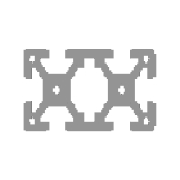
# Autodesk Inventor part: 615 mm
Saved by Autodesk Inventor 2016 (Build 200138000, 138)
## iProperties
IsCustomPart: 1
Created: 2023-12-03
Part Number: 615 mm
Material: Aluminum 6061
Description: ALU PROFILE 3060
Document SubType Name: Modeling
Standard: ALU PROFILE 3060
Designer: Riskinova Oktavia
Standard Revision: ALU PROFILE 3060
Manufacturer: ALU PROFILE 3060
Standards Organization: ALU PROFILE 3060
Language: en-US
Size Designation: (Unnamed 1)
Categories: <MemberInstance><Categories><Category DisplayName="Structural Shapes" InternalName="089c4875-fa83-4c05-b084-43b9cc11f5ed" Mnemonic="GRDR"><CategoryParameter DisplayName="Mass per Length Unit" InternalName="0bb95a10-148f-4027-a459-38d7b056702a" Mnemonic="shpmass"/><CategoryParameter DisplayName="Section Area" InternalName="1ff91680-64b0-4202-b9a3-7fd3f94bba3b" Mnemonic="secarea"/><CategoryParameter DisplayName="Radius of Gyration (x)" InternalName="25778675-03e9-40c1-b6a8-4a9ed693320d" Mnemonic="gyrradx"/><CategoryParameter DisplayName="Torsional Rigidity Modulus" InternalName="26c1ec35-5026-4c63-ad0a-751cf684a536" Mnemonic="torrigmod"/><CategoryParameter DisplayName="Distance of the Center of Gravity X-X" InternalName="26c9bdb8-9c79-4b4f-a92e-8e197583c9c4" Mnemonic="grcendistX"/><CategoryParameter DisplayName="Legacy Member ID" InternalName="340afe4f-75d7-48d3-ab7d-943f3c3da468" Mnemonic="LegacyMemberID"/><CategoryParameter DisplayName="Base Length" InternalName="42e34263-8f20-4d0e-ad48-bf1385b87c24" Mnemonic="shplen"/><CategoryParameter DisplayName="Moment of Inertia (y)" InternalName="4b9f58ea-bced-460e-81ea-3d29ca5a49e3" Mnemonic="inermomy"/><CategoryParameter DisplayName="Moment of Inertia (x)" InternalName="4cd780bc-73d7-43ac-917a-579e5cbd684d" Mnemonic="inermomx"/><CategoryParameter DisplayName="Custom Base Point" InternalName="4f1d1b73-316d-484b-a3df-9cbabb16eb77" Mnemonic="shpBasePoint"/><CategoryParameter DisplayName="Shape Height" InternalName="50274e7d-5ac0-4796-92cb-c59e54983c67" Mnemonic="shpheig"/><CategoryParameter DisplayName="Section Module (y)" InternalName="59eaa5e9-d227-48dc-b6c1-6920f96e0f95" Mnemonic="secmody"/><CategoryParameter DisplayName="Section Designation" InternalName="5a64d034-428d-49c8-ba32-7619764de20f" Mnemonic="shpdes"/><CategoryParameter DisplayName="Section Module (x)" InternalName="72cfad18-cf51-4ed4-aaa7-c6b224f8419f" Mnemonic="secmodx"/><CategoryParameter DisplayName="Torsional Section Modulus" InternalName="7c55a8dc-8844-49f9-a867-cc677b30ec9a" Mnemonic="torsecmod"/><CategoryParameter DisplayName="Shape Width" InternalName="7c717d54-a18f-4666-b4d4-573cce22c62c" Mnemonic="shpwdth"/><CategoryParameter DisplayName="Second Shape Thickness" InternalName="9251a8e1-85fd-4e47-af99-afdb762317d9" Mnemonic="shpthick2"/><CategoryParameter DisplayName="FG Authored" InternalName="9c666724-f362-4ea7-ac62-f6a007de5c69" Mnemonic="shpFGAuto"/><CategoryParameter DisplayName="Distance of the Center of Gravity Y-Y" InternalName="bcc4fb17-7af4-436a-8f8c-d0aa3b0248c5" Mnemonic="grcendistY"/><CategoryParameter DisplayName="Radius of Gyration (y)" InternalName="bfa18ebe-1636-4dbe-8d42-b263e0b73184" Mnemonic="gyrrady"/><CategoryParameter DisplayName="Shape Thickness" InternalName="d109cf76-8eb4-42fc-9800-4409734adc67" Mnemonic="shpthick"/><CategoryParameter DisplayName="Coefficient of Shear Displacement" InternalName="de4c90c6-aaa8-468f-a335-6737b311b5d3" Mnemonic="shdispc"/><Category DisplayName="Other" InternalName="f02205ff-2390-476f-921c-0b3185f88e84" Mnemonic="OTHSHP"><CategoryParameter DisplayName="Moment of Inertia (y)" InternalName="044c654e-f649-48ac-84cc-650a29ae31ca" Mnemonic="inermomy"/><CategoryParameter DisplayName="Shape Thickness" InternalName="12b1a788-9233-48fd-a933-2df8ff42b15f" Mnemonic="shpthick"/><CategoryParameter DisplayName="Mass per Length Unit" InternalName="2fd289d6-9394-4d2d-97e6-6659d7d4551d" Mnemonic="shpmass"/><CategoryParameter DisplayName="Radius of Gyration (y)" InternalName="743e1dfe-1bba-408b-b985-cf752b207386" Mnemonic="gyrrady"/><CategoryParameter DisplayName="Section Module (y)" InternalName="88b8bff9-a616-4028-93d5-ed4f79680d13" Mnemonic="secmody"/><CategoryParameter DisplayName="Section Area" InternalName="c46ecdf8-b6eb-4db9-8b25-30258930c1e3" Mnemonic="secarea"/><CategoryParameter DisplayName="Section Module (x)" InternalName="cac70804-9d39-43bb-be17-56ea1f39a6c2" Mnemonic="secmodx"/><CategoryParameter DisplayName="Moment of Inertia (x)" InternalName="ec6737bc-264f-43ed-b0bd-f6d410c2718d" Mnemonic="inermomx"/><CategoryParameter DisplayName="Radius of Gyration (x)" InternalName="ee72c61e-565e-4fd6-b448-66e1e1abcb7e" Mnemonic="gyrradx"/></Category></Category><Category DisplayName="DataType" InternalName="23b78d0f-2648-40c6-8793-ca6db495c9e8" Mnemonic="DATATYPE"><CategoryParameter DisplayName="DisplayName" InternalName="05415f3d-3907-474b-a020-eb9d644f4cf3" Mnemonic="DISPLAYNAME"/><CategoryParameter DisplayName="Standard" InternalName="0c0a119c-1e12-4c84-803f-101930972f5e" Mnemonic="STANDARD"/><CategoryParameter DisplayName="Description" InternalName="13903e3d-64b1-4950-80da-f627842ea37f" Mnemonic="DESCRIPTION"/><CategoryParameter DisplayName="Designation" InternalName="2675968c-4ce5-49e0-a4f5-552d29089031" Mnemonic="DESIGNATION"/><CategoryParameter DisplayName="Default Row" InternalName="2af9ec52-faaa-4026-b378-f9fa4afca842" Mnemonic="DEFAULTROW"/><CategoryParameter DisplayName="Folder Name" InternalName="3f06958e-8713-4116-9be7-ed6184ecc97b" Mnemonic="FOLDERNAME"/><CategoryParameter DisplayName="Revision Guid" InternalName="45a75005-10b1-4dfc-8d6d-dfe629f0b93c" Mnemonic="REVISIONGUID"/><CategoryParameter DisplayName="FileName" InternalName="8b46a4cc-9585-4fed-90c3-899f57e09a73" Mnemonic="FILENAME"/><CategoryParameter DisplayName="StdsOrg" InternalName="8f5914e1-4693-403f-8ab5-d37768198c9d" Mnemonic="STDSORG"/><CategoryParameter DisplayName="Family Version" InternalName="914462f6-6e19-4b14-ba84-155b9680b1d0" Mnemonic="FAMILYREVISION"/><CategoryParameter DisplayName="Standard Revision" InternalName="91d5a463-65c2-4fde-b823-3b7fea5e8e17" Mnemonic="STANDARDREVISION"/><CategoryParameter DisplayName="Member Revision" InternalName="a65d44b9-392f-4f4f-857b-e4b3d54996fe" Mnemonic="MEMBERREVISION"/><CategoryParameter DisplayName="ClipFormat" InternalName="bc51e27b-3422-4e78-93ef-cec197ddf230" Mnemonic="CLIPFORMAT"/><CategoryParameter DisplayName="Manufacturer" InternalName="cd6c7a72-a28a-4e50-99a9-2c7f4e13e5ad" Mnemonic="MANUFACTURER"/><CategoryParameter DisplayName="InternalName" InternalName="cf1d0246-76d9-4b4a-8305-fa0409afb5c1" Mnemonic="INTERNALNAME"/><CategoryParameter DisplayName="IsMetric" InternalName="e2385c5b-1ea4-4823-96a8-8de651266ec3" Mnemonic="ISMETRIC"/><Category DisplayName="Part" InternalName="c0e0b642-3bcb-4cc8-9e80-f96d35c4afa4" Mnemonic="PART"><CategoryParameter DisplayName="Part Number" InternalName="016b6077-bfbe-49bd-92c9-d8d59c39c941" Mnemonic="PARTNUMBER"/><CategoryParameter DisplayName="Stock Number" InternalName="4dba7c1c-e26c-444e-836c-b08b433409a8" Mnemonic="STOCKNUMBER"/><CategoryParameter DisplayName="Material Key" InternalName="5c9a8adb-dd2b-4535-b97f-0a94a95fe41f" Mnemonic="MATERIALKEY"/><CategoryParameter DisplayName="Material" InternalName="818a152a-d3c3-49ca-80ee-df7d91421b8e" Mnemonic="MATERIAL"/></Category></Category></Categories><FamilyTemplate Id="i profile 30x60"><FamilyTemplateParameters><FamilyTemplateParameter ObjectType="kUserParameterObject" ValueType="xs:double" Id="1" ObjectReferenceKey="LENGTH"/><FamilyTemplateParameter ObjectType="kUserParameterObject" ValueType="xs:double" Id="3" ObjectReferenceKey="X"/><FamilyTemplateParameter ObjectType="kPartComponentDefinitionObject" ValueType="xs:string" Id="5" SubObjectId="Material"/><FamilyTemplateParameter ObjectType="kPropertyObject" ValueType="xs:string" Id="17" ObjectReferenceKey="{32853F0F-3444-11d1-9E93-0060B03C1CA6}" SubObjectId="5"/><FamilyTemplateParameter ObjectType="kPropertyObject" ValueType="xs:string" Id="18" ObjectReferenceKey="{32853F0F-3444-11d1-9E93-0060B03C1CA6}" SubObjectId="52"/></FamilyTemplateParameters></FamilyTemplate><CategoryParameterMap><ParamToTemplateMap><ParamToTemplate CategoryParameter="//CategoryParameter[@InternalName='cf1d0246-76d9-4b4a-8305-fa0409afb5c1']" ConstantValue="567a99e7-1936-4fa4-9c8c-24f894b82731"/><ParamToTemplate CategoryParameter="//CategoryParameter[@InternalName='45a75005-10b1-4dfc-8d6d-dfe629f0b93c']" ConstantValue="4680624b-5eff-4c3e-a2a1-f8e39fc0d9b8"/><ParamToTemplate CategoryParameter="//CategoryParameter[@InternalName='3f06958e-8713-4116-9be7-ed6184ecc97b']" ConstantValue="ALU PROFILE 3060"/><ParamToTemplate CategoryParameter="//CategoryParameter[@InternalName='8f5914e1-4693-403f-8ab5-d37768198c9d']" ConstantValue="ALU PROFILE 3060"/><ParamToTemplate CategoryParameter="//CategoryParameter[@InternalName='0c0a119c-1e12-4c84-803f-101930972f5e']" ConstantValue="ALU PROFILE 3060"/><ParamToTemplate CategoryParameter="//CategoryParameter[@InternalName='91d5a463-65c2-4fde-b823-3b7fea5e8e17']" ConstantValue="ALU PROFILE 3060"/><ParamToTemplate CategoryParameter="//CategoryParameter[@InternalName='cd6c7a72-a28a-4e50-99a9-2c7f4e13e5ad']" ConstantValue="ALU PROFILE 3060"/><ParamToTemplate CategoryParameter="//CategoryParameter[@InternalName='13903e3d-64b1-4950-80da-f627842ea37f']" ConstantValue="ALU PROFILE 3060"/><ParamToTemplate CategoryParameter="//CategoryParameter[@InternalName='05415f3d-3907-474b-a020-eb9d644f4cf3']" ConstantValue="ALU PROFILE 3060"/><ParamToTemplate CategoryParameter="//CategoryParameter[@InternalName='914462f6-6e19-4b14-ba84-155b9680b1d0']" ConstantValue="11"/><ParamToTemplate CategoryParameter="//CategoryParameter[@InternalName='bc51e27b-3422-4e78-93ef-cec197ddf230']" ConstantValue="CF_INVENTOR.STDPARTS"/><ParamToTemplate CategoryParameter="//CategoryParameter[@InternalName='e2385c5b-1ea4-4823-96a8-8de651266ec3']" ConstantValue="true"/><ParamToTemplate CategoryParameter="//CategoryParameter[@InternalName='2af9ec52-faaa-4026-b378-f9fa4afca842']" ConstantValue="1"/><ParamToTemplate CategoryParameter="//CategoryParameter[@InternalName='9c666724-f362-4ea7-ac62-f6a007de5c69']" ConstantValue="1"/><ParamToTemplate CategoryParameter="//CategoryParameter[@InternalName='8b46a4cc-9585-4fed-90c3-899f57e09a73']" ConstantValue="i profile 30x60-01"/><ParamToTemplate CategoryParameter="//CategoryParameter[@InternalName='a65d44b9-392f-4f4f-857b-e4b3d54996fe']" ConstantValue="193b8da3-a0ee-4455-b78a-0fc36cc979fc"/><ParamToTemplate CategoryParameter="//CategoryParameter[@InternalName='a65d44b9-392f-4f4f-857b-e4b3d54996fe']" ConstantValue="193b8da3-a0ee-4455-b78a-0fc36cc979fc"/><ParamToTemplate CategoryParameter="//CategoryParameter[@InternalName='2675968c-4ce5-49e0-a4f5-552d29089031']" TemplateParameter="18"/><ParamToTemplate CategoryParameter="//CategoryParameter[@InternalName='42e34263-8f20-4d0e-ad48-bf1385b87c24']" TemplateParameter="1"/><ParamToTemplate CategoryParameter="//CategoryParameter[@InternalName='818a152a-d3c3-49ca-80ee-df7d91421b8e']" TemplateParameter="5"/><ParamToTemplate CategoryParameter="//CategoryParameter[@InternalName='016b6077-bfbe-49bd-92c9-d8d59c39c941']" TemplateParameter="17"/></ParamToTemplateMap></CategoryParameterMap></MemberInstance>
Density: 2.7 g/cm^3
Appearance: Aluminum - Flat
_CCFamilyMember: 1
_CCFamilyDisplayName: ALU PROFILE 3060 - ALU PROFILE 3060
_FrameMemberDoc: Frame Member File
_Version: 15.0.0
_GetPNFromCC: 1
X: 30.000 mm
LENGTH: 450.000 mm
G_W: 60.000 mm
G_H: 30.000 mm
+3EE16979-5328-4CA1-8470-071E4131E1F0+CUTDETAIL1: Cut
G_L: 615.000 mm
Author: Riskinova Oktavia
Autodesk Inventor part; units mm, degrees
ref_plane "Start Plane" through (0, 0, -180) normal (0, 0, 1) x (1, 0, 0)
ref_plane "End Plane" through (0, 0, 435) normal (0, 0, 1) x (1, 0, 0)
sketch "Sketch" plane through (0, 0, 0) normal (0, 0, 1) x (1, 0, 0)
  line L0 (-30, 15) -> (0, -15) construction
  line L1 (0, 15) -> (-30, -15) construction
  line L2 (-20.2, 15) -> (-20.2, 14.2)
  line L3 (-20.2, 14.2) -> (-19.1, 14.2)
  line L4 (-19.1, 14.2) -> (-19.1, 12.2)
  line L5 (-19.1, 12.2) -> (-23.25, 12.2)
  line L6 (-23.25, 12.2) -> (-23.25, 10.2)
  line L7 (-23.25, 10.2) -> (-18.85, 5.8)
  line L8 (-18.85, 5.8) -> (-11.15, 5.8)
  line L9 (-6.75, 12.2) -> (-10.9, 12.2)
  line L10 (-10.9, 12.2) -> (-10.9, 14.2)
  line L11 (-10.9, 14.2) -> (-9.8, 14.2)
  line L12 (-9.8, 14.2) -> (-9.8, 15)
  line L13 (-6.75, 12.2) -> (-6.75, 10.2)
  line L14 (-6.75, 10.2) -> (-11.15, 5.8)
  line L15 (-20.2, -15) -> (-20.2, -14.2)
  line L16 (-20.2, -14.2) -> (-19.1, -14.2)
  line L17 (-19.1, -14.2) -> (-19.1, -12.2)
  line L18 (-19.1, -12.2) -> (-23.25, -12.2)
  line L19 (-23.25, -12.2) -> (-23.25, -10.2)
  line L20 (-23.25, -10.2) -> (-18.85, -5.8)
  line L21 (-18.85, -5.8) -> (-11.15, -5.8)
  line L22 (-6.75, -10.2) -> (-11.15, -5.8)
  line L23 (-6.75, -12.2) -> (-6.75, -10.2)
  line L24 (-6.75, -12.2) -> (-10.9, -12.2)
  line L25 (-10.9, -12.2) -> (-10.9, -14.2)
  line L26 (-10.9, -14.2) -> (-9.8, -14.2)
  line L27 (-9.8, -14.2) -> (-9.8, -15)
  line L28 (-2.8, -8.25) -> (-4.8, -8.25)
  line L29 (-4.8, -8.25) -> (-9.2, -3.85)
  line L30 (-9.2, -3.85) -> (-9.2, 3.85)
  line L31 (-9.2, 3.85) -> (-4.8, 8.25)
  line L32 (-4.8, 8.25) -> (-2.8, 8.25)
  line L33 (-30, 5.2) -> (-29.2, 5.2)
  line L34 (-29.2, 5.2) -> (-29.2, 4.1)
  line L35 (-29.2, 4.1) -> (-27.2, 4.1)
  line L36 (-27.2, 4.1) -> (-27.2, 8.25)
  line L37 (-25.2, 8.25) -> (-27.2, 8.25)
  line L38 (-20.8, 3.85) -> (-25.2, 8.25)
  line L39 (-20.8, -3.85) -> (-20.8, 3.85)
  line L40 (-25.2, -8.25) -> (-20.8, -3.85)
  line L41 (-27.2, -4.1) -> (-27.2, -8.25)
  line L42 (-29.2, -4.1) -> (-27.2, -4.1)
  line L43 (-29.2, -5.2) -> (-29.2, -4.1)
  line L44 (-30, -5.2) -> (-29.2, -5.2)
  line L45 (-27.2, -8.25) -> (-25.2, -8.25)
  circle A0 centre (-26.5, 11.5) radius 1.65
  circle A1 centre (-26.5, -11.5) radius 1.65
  line L46 (-30, -13) -> (-30, -5.2)
  line L47 (-30, 5.2) -> (-30, 13)
  line L48 (-20.2, -15) -> (-28, -15)
  line L49 (0, 15) -> (30, -15) construction
  line L50 (30, 15) -> (0, -15) construction
  line L51 (9.8, 15) -> (9.8, 14.2)
  line L52 (9.8, 14.2) -> (10.9, 14.2)
  line L53 (10.9, 14.2) -> (10.9, 12.2)
  line L54 (10.9, 12.2) -> (6.75, 12.2)
  line L55 (6.75, 12.2) -> (6.75, 10.2)
  line L56 (6.75, 10.2) -> (11.15, 5.8)
  line L57 (11.15, 5.8) -> (18.85, 5.8)
  line L58 (23.25, 12.2) -> (19.1, 12.2)
  line L59 (19.1, 12.2) -> (19.1, 14.2)
  line L60 (19.1, 14.2) -> (20.2, 14.2)
  line L61 (20.2, 14.2) -> (20.2, 15)
  line L62 (23.25, 12.2) -> (23.25, 10.2)
  line L63 (23.25, 10.2) -> (18.85, 5.8)
  line L64 (9.8, -15) -> (9.8, -14.2)
  line L65 (9.8, -14.2) -> (10.9, -14.2)
  line L66 (10.9, -14.2) -> (10.9, -12.2)
  line L67 (10.9, -12.2) -> (6.75, -12.2)
  line L68 (6.75, -12.2) -> (6.75, -10.2)
  line L69 (6.75, -10.2) -> (11.15, -5.8)
  line L70 (11.15, -5.8) -> (18.85, -5.8)
  line L71 (23.25, -10.2) -> (18.85, -5.8)
  line L72 (23.25, -12.2) -> (23.25, -10.2)
  line L73 (23.25, -12.2) -> (19.1, -12.2)
  line L74 (19.1, -12.2) -> (19.1, -14.2)
  line L75 (19.1, -14.2) -> (20.2, -14.2)
  line L76 (20.2, -14.2) -> (20.2, -15)
  line L77 (30, 5.2) -> (29.2, 5.2)
  line L78 (29.2, 5.2) -> (29.2, 4.1)
  line L79 (29.2, 4.1) -> (27.2, 4.1)
  line L80 (27.2, 4.1) -> (27.2, 8.25)
  line L81 (30, -5.2) -> (29.2, -5.2)
  line L82 (29.2, -5.2) -> (29.2, -4.1)
  line L83 (29.2, -4.1) -> (27.2, -4.1)
  line L84 (27.2, -4.1) -> (27.2, -8.25)
  line L85 (27.2, -8.25) -> (25.2, -8.25)
  line L86 (25.2, -8.25) -> (20.8, -3.85)
  line L87 (20.8, -3.85) -> (20.8, 3.85)
  line L88 (20.8, 3.85) -> (25.2, 8.25)
  line L89 (25.2, 8.25) -> (27.2, 8.25)
  line L90 (4.8, 8.25) -> (2.8002, 8.25)
  line L91 (9.2, 3.85) -> (4.8, 8.25)
  line L92 (9.2, -3.85) -> (9.2, 3.85)
  line L93 (4.8, -8.25) -> (9.2, -3.85)
  line L94 (2.8, -8.25) -> (4.8, -8.25)
  circle A2 centre (26.5, 11.5) radius 1.65
  circle A3 centre (26.5, -11.5) radius 1.65
  line L95 (28, -15) -> (20.2, -15)
  circle A4 centre (-15, 0) radius 2
  circle A5 centre (15, 0) radius 2
  line L96 (-2.8, 8.25) -> (-2.8, 12.2)
  line L97 (2.8002, 8.25) -> (2.8002, 12.2)
  line L98 (2.8002, 12.2) -> (-2.8, 12.2)
  line L99 (-2.8, -8.25) -> (-2.8, -12.2)
  line L100 (-2.8, -12.2) -> (2.8, -12.2)
  line L101 (2.8, -12.2) -> (2.8, -8.25)
  line L102 (30, 13) -> (30, 5.2)
  line L103 (30, -5.2) -> (30, -13)
  arc A6 (-28, 15) -> (-30, 13) centre (-28, 13) ccw
  arc A7 (30, 13) -> (28, 15) centre (28, 13) ccw
  arc A8 (28, -15) -> (30, -13) centre (28, -13) ccw
  arc A9 (-30, -13) -> (-28, -15) centre (-28, -13) ccw
  line L104 (-28, 15) -> (-20.2, 15)
  line L105 (20.2, 15) -> (28, 15)
  line L106 (-9.8, -15) -> (9.8, -15)
  line L107 (-9.8, 15) -> (9.8, 15)
  point P0 (0, 0)
  point P1 (-15, 0)
  point P2 (-15, 0)
  point P3 (15, 0)
  point P4 (15, 0)
  point P5 (0, -15)
  dimension "d0" = 8.2
  dimension "d2" = 10.4
  dimension "d7" = 16.5
  dimension "d9" = 0.8
  dimension "d10" = 2
  dimension "d11" = 2
  dimension "d20" = 2
  dimension "d27" = 8.2
  dimension "d29" = 10.4
  dimension "d34" = 16.5
  dimension "d36" = 0.8
  dimension "d37" = 2
  dimension "d38" = 2
  dimension "d39" = 0.8
  dimension "d40" = 10.4
  dimension "d42" = 8.2
  dimension "d44" = 2
  dimension "d45" = 16.5
  dimension "d47" = 2
  dimension "d49" = 23
  dimension "d50" = 11.5
  dimension "d52" = 11.5
  dimension "d53" = 3.3
  dimension "d54" = 10.9
  dimension "d56" = 7.7
  dimension "d58" = 18.4
  dimension "d59" = 90
  dimension "d63" = 135
  dimension "d64" = 3.5
  dimension "d65" = 4
  dimension "d75" = 0.8
  dimension "d76" = 1.1
  dimension "d77" = 2
  dimension "d78" = 4.4
  dimension "d82" = 0.8
  dimension "d83" = 8.2
  dimension "d84" = 8.2
  dimension "d85" = 0.8
  dimension "d86" = 1.1
  dimension "d87" = 2
  dimension "d88" = 1.1
  dimension "d89" = 0.8
  dimension "d90" = 4.15
  dimension "d91" = 4.15
  dimension "d94" = 4.4
  dimension "d95" = 6.4
  dimension "d96" = 4.4
  dimension "d97" = 3.85
  dimension "d98" = 45
  dimension "d99" = 4.1
  dimension "d100" = 8.25
  dimension "d101" = 4.1
  dimension "d102" = 6.3
  dimension "d103" = 3.3
  dimension "d105" = 2
  dimension "d106" = 2.7577
  dimension "d107" = 6.2225
  dimension "d108" = 3.25
  dimension "d109" = 4.1
  dimension "d110" = 5.2
  dimension "d111" = 5.8
  dimension "d112" = 2.7577
  dimension "d113" = 2.7577
  dimension "d114" = 6.2225
  constraints: 216 end point, 24 perpendicular, 22 point on line, 16 parallel, 10 centre point, 8 horizontal, 8 midpoint, 8 point on circle, 8 tangent, 7 vertical, 6 equal radius, 5 vertical alignment, 2 coincident, 2 collinear, 1 horizontal alignment
  measures "d0" distance between parallel lines of L10 L4
  measures "d2" distance from line of L12.start L2
  measures "d7" distance between parallel lines of L6 L13
  measures "d9" distance of L12.start L12.end
  measures "d10" distance of L10.start L10.end
  measures "d11" distance of L9.start L14.start
  measures "d20" distance of L28.start L28.end
  measures "d27" distance between parallel lines of L59 L53
  measures "d29" distance from line of L61.start L51
  measures "d34" distance between parallel lines of L55 L62
  measures "d36" distance of L61.start L61.end
  measures "d37" distance of L59.start L59.end
  measures "d38" distance of L58.start L63.start
  measures "d39" distance of L81.start L82.start
  measures "d40" distance between parallel lines of L81 L77
  measures "d42" distance between parallel lines of L79 L83
  measures "d44" distance of L82.end L83.end
  measures "d45" distance of L80.end L84.end
  measures "d47" distance of L84.end L85.end
  measures "d49" distance of A3.centre A2.centre
  measures "d50" horizontal distance of point (15, 0) A3.centre
  measures "d52" horizontal distance of point (15, 0) A3.centre
  measures "d53" diameter of A3
  measures "d54" distance between parallel lines of L17 L46
  measures "d56" distance of L21.start L21.end
  measures "d58" distance between parallel lines of L30 L92
  measures "d59" angle of L63 L56
  measures "d63" angle of L0 L47
  measures "d64" distance from line of A1.centre L46
  measures "d65" diameter of A5
  measures "d75" distance of L33.start L34.start
  measures "d76" distance of L34.start L35.start
  measures "d77" distance of L35.start L36.start
  measures "d78" horizontal distance of L38.start L38.end
  measures "d82" distance of L26.end L27.end
  measures "d83" distance between parallel lines of L17 L25
  measures "d84" distance between parallel lines of L74 L66
  measures "d85" distance of L64.start L64.end
  measures "d86" distance of L64.end L65.end
  measures "d87" distance of L73.end L74.end
  measures "d88" distance of L74.end L75.end
  measures "d89" distance of L75.end L76.end
  measures "d90" distance of L66.end L67.end
  measures "d91" distance of L72.start L73.end
  measures "d94" horizontal distance of L68.end L70.start
  measures "d95" distance between parallel lines of L67 L70
  measures "d96" horizontal distance of L68.end L70.start
  measures "d97" horizontal distance of point (15, 0) L70.start
  measures "d98" angle of L1 L4
  measures "d99" distance from line of point (-15, 0) L4
  measures "d100" distance from line of point (-15, 0) L13
  measures "d101" distance from line of point (-15, 0) L10
  measures "d102" distance from line of A0.centre L2
  measures "d103" diameter of A0
  measures "d105" distance of L38.end L37.end
  measures "d106" distance between parallel lines of L7 L38
  measures "d107" distance of L7.start L8.start
  measures "d108" distance from line of L37 A0.centre
  measures "d109" distance from line of point (-15, 0) L35
  measures "d110" distance from line of point (-15, 0) L33
  measures "d111" distance from line of point (-15, 0) L39
  measures "d112" distance between parallel lines of L14 L31
  measures "d113" distance between parallel lines of L56 L91
  measures "d114" distance of L93.start L92.start
extrude "Body" add sketch "Sketch" along normal up to surface (615 mm away) from surface at -180
sketch "Sketch4" plane through (0, 0, 0) normal (0, 0, 1) x (1, 0, 0)
  line L0 (0, 0) -> (10, 0)
ref_plane "Work Plane3" through (0, 0, 0) normal (0, -1, 0) x (1, 0, 0)
sketch "Sketch5" plane through (0, 0, 0) normal (0, -1, 0) x (1, 0, 0)
  line L0 (-2, -180) -> (12, -180)
  line L1 (-2, 435) -> (12, 435)
  dimension "d178" = 615
  measures "d178" distance between parallel lines of L0 L1
ref_plane "Work Plane4" through (-370, -13, 435) normal (0, 0, 1) x (1, 0, 0)
split "Split1" plane through (-370, -13, 435) removes the side toward (0, 0, 1)
equation "\"d50\" = 0.5 * d49"
equation "\"d52\" = 0.5 * d51"
equation "\"G_OFFSET_END\" = -15"
equation "\"G_L\" = 615"
equation "\"d51\" = 23"
body "Solid2"
